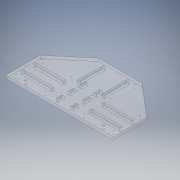
# Autodesk Inventor part: phone_holder_back
Saved by Autodesk Inventor 2019 (Build 230136000, 136)
## iProperties
Created: 2019-02-17
Part Number: phone_holder_back
Material: Acrylic, Clear
Document SubType Name: Modeling
Designer: suchanek
Density: 1.19 g/cm^3
Appearance: Transparent - Clear
Author: suchanek
Autodesk Inventor part; units mm, degrees
ref_plane "YZ Plane" through (0, 0, 0) normal (1, 0, 0) x (0, 1, 0)
ref_plane "XZ Plane" through (0, 0, 0) normal (0, 1, 0) x (-1, 0, 0)
ref_plane "XY Plane" through (0, 0, 0) normal (0, 0, 1) x (1, 0, 0)
sketch "Sketch2" plane through (0, 0, 0) normal (0, 1, 0) x (-1, 0, 0)
  line L0 (110, 62.5) -> (-110, 62.5)
  line L1 (-110, 62.5) -> (-110, -62.5)
  line L2 (-110, -62.5) -> (110, -62.5)
  line L3 (110, -62.5) -> (110, 62.5)
  line L4 (110, 62.5) -> (-110, -62.5) construction
  line L5 (-110, 62.5) -> (110, -62.5) construction
  line L6 (12.4, -7.5) -> (17.5, -7.5)
  line L7 (17.5, -7.5) -> (17.5, 4.2)
  line L8 (17.5, 4.2) -> (12.4, 4.2)
  line L9 (12.4, 4.2) -> (12.4, -7.5)
  line L10 (12.4, 16.5) -> (17.5, 16.5)
  line L11 (17.5, 16.5) -> (17.5, 28.2)
  line L12 (17.5, 28.2) -> (12.4, 28.2)
  line L13 (12.4, 28.2) -> (12.4, 16.5)
  line L14 (12.4, 40.5) -> (17.5, 40.5)
  line L15 (17.5, 40.5) -> (17.5, 52.2)
  line L16 (17.5, 52.2) -> (12.4, 52.2)
  line L17 (12.4, 52.2) -> (12.4, 40.5)
  line L18 (-17.5, -7.5) -> (-12.4, -7.5)
  line L19 (-12.4, -7.5) -> (-12.4, 4.2)
  line L20 (-12.4, 4.2) -> (-17.5, 4.2)
  line L21 (-17.5, 4.2) -> (-17.5, -7.5)
  line L22 (-17.5, 16.5) -> (-12.4, 16.5)
  line L23 (-12.4, 16.5) -> (-12.4, 28.2)
  line L24 (-12.4, 28.2) -> (-17.5, 28.2)
  line L25 (-17.5, 28.2) -> (-17.5, 16.5)
  line L26 (-17.5, 40.5) -> (-12.4, 40.5)
  line L27 (-12.4, 40.5) -> (-12.4, 52.2)
  line L28 (-12.4, 52.2) -> (-17.5, 52.2)
  line L29 (-17.5, 52.2) -> (-17.5, 40.5)
  line L30 (0, 0) -> (0, -18.9718)
  line L31 (25, -2.5) -> (25, -52.5) construction
  line L32 (22.45, -2.5) -> (22.45, -52.5)
  line L33 (27.55, -52.5) -> (27.55, -2.5)
  arc A0 (27.55, -2.5) -> (22.45, -2.5) centre (25, -2.5) ccw
  arc A1 (22.45, -52.5) -> (27.55, -52.5) centre (25, -52.5) ccw
  line L34 (100, 12.5) -> (40, 12.5) construction
  line L35 (100, 15.05) -> (40, 15.05)
  line L36 (40, 9.95) -> (100, 9.95)
  arc A2 (100, 9.95) -> (100, 15.05) centre (100, 12.5) ccw
  arc A3 (40, 15.05) -> (40, 9.95) centre (40, 12.5) ccw
  line L37 (100, 37.5) -> (40, 37.5) construction
  line L38 (100, 40.05) -> (40, 40.05)
  line L39 (40, 34.95) -> (100, 34.95)
  arc A4 (100, 34.95) -> (100, 40.05) centre (100, 37.5) ccw
  arc A5 (40, 40.05) -> (40, 34.95) centre (40, 37.5) ccw
  line L40 (-25, -2.5) -> (-25, -52.5) construction
  line L41 (-22.45, -2.5) -> (-22.45, -52.5)
  line L42 (-27.55, -52.5) -> (-27.55, -2.5)
  arc A6 (-22.45, -2.5) -> (-27.55, -2.5) centre (-25, -2.5) ccw
  arc A7 (-27.55, -52.5) -> (-22.45, -52.5) centre (-25, -52.5) ccw
  line L43 (-100, 12.5) -> (-40, 12.5) construction
  line L44 (-100, 15.05) -> (-40, 15.05)
  line L45 (-40, 9.95) -> (-100, 9.95)
  arc A8 (-100, 15.05) -> (-100, 9.95) centre (-100, 12.5) ccw
  arc A9 (-40, 9.95) -> (-40, 15.05) centre (-40, 12.5) ccw
  line L46 (-100, 37.5) -> (-40, 37.5) construction
  line L47 (-100, 40.05) -> (-40, 40.05)
  line L48 (-40, 34.95) -> (-100, 34.95)
  arc A10 (-100, 40.05) -> (-100, 34.95) centre (-100, 37.5) ccw
  arc A11 (-40, 34.95) -> (-40, 40.05) centre (-40, 37.5) ccw
  circle A12 centre (80, 52.5) radius 2.25
  circle A13 centre (-80, 52.5) radius 2.25
  line L49 (110, -7.5) -> (45, -62.5)
  line L50 (-45, -62.5) -> (-110, -7.5)
  circle A14 centre (100, 52.5) radius 0.9
  circle A15 centre (40, -52.5) radius 0.9
  circle A16 centre (100, -2.5) radius 0.9
  circle A17 centre (40, -2.5) radius 0.9
  circle A18 centre (40, 52.5) radius 0.9
  circle A19 centre (-100, 52.5) radius 0.9
  circle A20 centre (-40, -52.5) radius 0.9
  circle A21 centre (-100, -2.5) radius 0.9
  circle A22 centre (-40, -2.5) radius 0.9
  circle A23 centre (-40, 52.5) radius 0.9
  circle A24 centre (14.95, 10.35) radius 1.125
  circle A25 centre (-14.95, 10.35) radius 1.125
  point P0 (25, -27.5)
  point P1 (70, 12.5)
  point P2 (70, 37.5)
  point P3 (-25, -27.5)
  point P4 (-70, 12.5)
  point P5 (-70, 37.5)
  dimension "d52" = 220
  dimension "d53" = 125
  dimension "d54" = 11.7
  dimension "d55" = 5.1
  dimension "d58" = 24
  dimension "d61" = 29.9
  dimension "d65" = 55
  dimension "d66" = 5.1
  dimension "d68" = 100
  dimension "d69" = 115
  dimension "d70" = 40
  dimension "d71" = 65
  dimension "d72" = 15
  dimension "d73" = 25
  dimension "d75" = 15
  dimension "d76" = 4.5
  dimension "d79" = 30
  dimension "d80" = 10
  dimension "d81" = 20
  dimension "d82" = 20
  dimension "d83" = 1.8
  dimension "d84" = 1.8
  dimension "d85" = 1.8
  dimension "d86" = 1.8
  dimension "d87" = 1.8
  dimension "d88" = 2.25
  dimension "d89" = 2.55
  dimension "d90" = 6.15
  constraints: 114 end point, 29 symmetric about line, 26 centre point, 24 point on circle, 12 tangent, 8 parallel, 7 vertical alignment, 6 horizontal alignment, 5 midpoint, 4 point on line, 3 horizontal, 3 perpendicular, 3 vertical, 2 equal radius, 54 other
  measures "d52" distance of L2.end L1.end
  measures "d53" distance of L1.end L0.end
  measures "d54" distance of L8.end L6.start
  measures "d55" distance of L6.start L6.end
  measures "d58" distance of L6.start L10.start
  measures "d61" distance of L6.start L18.start
  measures "d65" distance between parallel lines of L2 L6
  measures "d66" diameter of A1
  measures "d68" distance from line of L30 L34.start
  measures "d69" distance from line of L0 L31.end
  measures "d70" distance from line of L30 L34.end
  measures "d71" distance from line of L0 L31.start
  measures "d72" horizontal distance of L31.start L34.end
  measures "d73" distance from line of L0 L37.end
  measures "d75" horizontal distance of L31.start L34.end
  measures "d76" diameter of A12
  measures "d79" distance from line of L3 A12.centre
  measures "d80" distance from line of L0 A12.centre
  measures "d81" distance from line of L49.end L31
  measures "d82" distance from line of L49.start L34
  measures "d83" diameter of A14
  measures "d84" diameter of A15
  measures "d85" diameter of A16
  measures "d86" diameter of A17
  measures "d87" diameter of A18
  measures "d88" diameter of A24
  measures "d89" distance from line of L13 A24.centre
  measures "d90" distance from line of L10 A24.centre
extrude "Extrusion2" add sketch "Sketch2" along normal blind 6 contours L3 L49 L2 L50 L1 L0
body "Solid2"
